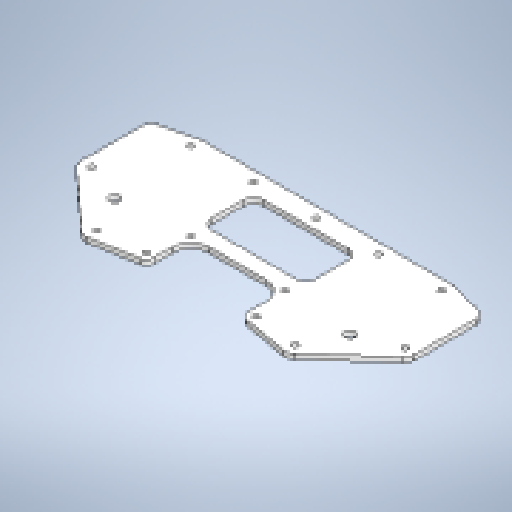
# Autodesk Inventor part: Chassis
Saved by Autodesk Inventor 2023.1 (Build 271208000, 208)
## iProperties
Created: 2022-05-26
Part Number: Chassis
Material: UHMW, White
Document SubType Name: Modeling
Designer: Nathan Cai
Density: 0.94 g/cm^3
Appearance: Smooth - White
Mass: 17.5924 g
Surface Area: 250.439 cm^2
Volume: 18.7153 cm^3
Author: Nathan Cai
Autodesk Inventor part; units mm, degrees
ref_plane "YZ Plane" through (0, 0, 0) normal (1, 0, 0) x (0, 1, 0)
ref_plane "XZ Plane" through (0, 0, 0) normal (0, 1, 0) x (-1, 0, 0)
ref_plane "XY Plane" through (0, 0, 0) normal (0, 0, 1) x (1, 0, 0)
sketch "Sketch1" plane through (0, 0, 0) normal (0, 1, 0) x (-1, 0, 0)
  line L0 (101.6, 38.1) -> (-101.6, 38.1) construction
  line L1 (-101.6, 38.1) -> (-101.6, -38.1) construction
  line L2 (-101.6, -38.1) -> (101.6, -38.1) construction
  line L3 (101.6, -38.1) -> (101.6, 38.1) construction
  line L4 (101.6, 38.1) -> (-101.6, -38.1) construction
  line L5 (-101.6, 38.1) -> (101.6, -38.1) construction
  line L6 (-28.575, 66.675) -> (28.575, 66.675) construction
  line L7 (28.575, 66.675) -> (28.575, 9.525)
  line L8 (28.575, 9.525) -> (-28.575, 9.525) construction
  line L9 (-28.575, 9.525) -> (-28.575, 66.675)
  line L10 (-28.575, 66.675) -> (28.575, 9.525) construction
  line L11 (28.575, 66.675) -> (-28.575, 9.525) construction
  circle A0 centre (-38.1, 50.8) radius 3.175
  line L12 (0, 38.1) -> (0, -38.1) construction
  circle A1 centre (-38.1, 50.8) radius 9.525
  line L13 (-38.1, 60.325) -> (-28.575, 60.325)
  circle A2 centre (38.1, 50.8) radius 3.175
  circle A3 centre (38.1, 50.8) radius 9.525
  line L14 (38.1, 60.325) -> (28.575, 60.325)
  circle A4 centre (-76.2, -38.1) radius 1.7526
  circle A5 centre (-95.25, 3.175) radius 1.7526
  circle A6 centre (76.2, -38.1) radius 1.7526
  circle A7 centre (95.25, 3.175) radius 1.7526
  line L15 (-101.6, -38.1) -> (-101.6, 6.35)
  line L16 (-101.6, 6.35) -> (-44.4797, 57.8728)
  line L17 (101.6, -38.1) -> (101.6, 6.35)
  line L18 (101.6, 6.35) -> (44.4797, 57.8728)
  line L19 (-42.6417, 42.4275) -> (-87.975, 1.5367) construction
  line L20 (-87.975, 1.5367) -> (-87.975, -38.1)
  line L21 (87.975, -38.1) -> (87.975, 1.5367)
  line L22 (87.975, 1.5367) -> (42.6417, 42.4275) construction
  line L23 (0, -38.1) -> (-95.25, -38.1) construction
  line L24 (0, -38.1) -> (95.25, -38.1) construction
  circle A8 centre (-60.325, 35.0287) radius 1.7526
  circle A9 centre (-33.3375, 31.75) radius 1.7526
  line L25 (-38.1, 0) -> (-38.1, 41.275)
  line L26 (-38.1, 0) -> (0, 0) construction
  circle A10 centre (60.325, 35.0287) radius 1.7526
  circle A11 centre (33.3375, 31.75) radius 1.7526
  line L27 (38.1, 0) -> (38.1, 41.275)
  line L28 (38.1, 0) -> (0, 0) construction
  line L29 (-87.975, 0) -> (-65.115, 0)
  line L30 (-65.115, 0) -> (-65.115, -31.75)
  line L31 (-65.115, -31.75) -> (-87.975, -31.75)
  line L32 (-101.6, -38.1) -> (101.6, -38.1) construction
  line L33 (101.6, -38.1) -> (101.6, 19.05)
  line L34 (101.6, 19.05) -> (-101.6, 19.05) construction
  line L35 (-101.6, 19.05) -> (-101.6, -38.1)
  line L36 (-101.6, 19.05) -> (-87.5203, 19.05) construction
  line L37 (87.5203, 19.05) -> (101.6, 19.05) construction
  circle A12 centre (-38.1, 0) radius 3.175 construction
  circle A13 centre (-38.1, 0) radius 6.35 construction
  circle A14 centre (38.1, 0) radius 3.175 construction
  circle A15 centre (38.1, 0) radius 6.35 construction
  circle A16 centre (28.575, 9.525) radius 1.7526
  circle A17 centre (28.575, 9.525) radius 4.7625
  arc A18 (17.0773, 9.525) -> (28.575, 21.0227) centre (17.0773, 21.0227) ccw
  circle A19 centre (-28.575, 9.525) radius 1.7526
  circle A20 centre (-28.575, 9.525) radius 4.7625
  arc A21 (-28.575, 21.0227) -> (-17.0773, 9.525) centre (-17.0773, 21.0227) ccw
  arc A22 (31.4325, 5.715) -> (38.1, 19.05) centre (21.4312, 19.05) ccw
  arc A23 (-38.1, 19.05) -> (-31.4325, 5.715) centre (-21.4312, 19.05) ccw
  line L38 (-61.94, -38.1) -> (-61.94, 25.0204)
  line L39 (87.975, 0) -> (65.115, 0)
  line L40 (65.115, 0) -> (65.115, -31.75)
  line L41 (65.115, -31.75) -> (87.975, -31.75)
  line L42 (61.94, -38.1) -> (61.94, 25.0204)
  line L43 (-28.575, 4.7625) -> (28.575, 4.7625)
  line L44 (101.6, -31.75) -> (-101.6, -31.75)
  line L45 (-101.6, -31.75) -> (-101.6, -44.45) construction
  line L46 (-101.6, -44.45) -> (101.6, -44.45)
  line L47 (101.6, -44.45) -> (101.6, -31.75) construction
  circle A24 centre (0, -38.1) radius 1.7526
  circle A25 centre (38.1, -38.1) radius 1.7526
  circle A26 centre (-38.1, -38.1) radius 1.7526
  line L48 (101.6, -38.1) -> (76.2, -44.45)
  line L49 (-101.6, -38.1) -> (-76.2, -44.45)
  line L50 (76.2, -38.1) -> (76.2, -44.45) construction
  line L51 (-76.2, -38.1) -> (-76.2, -44.45) construction
  line L52 (59.1924, 41.2769) -> (32.488, 36.4361)
  circle A27 centre (60.325, 35.0287) radius 6.35
  circle A28 centre (33.3375, 31.75) radius 4.7625
  line L53 (-59.1924, 41.2769) -> (-32.488, 36.4361)
  circle A29 centre (-60.325, 35.0287) radius 6.35
  circle A30 centre (-33.3375, 31.75) radius 4.7625
  line L54 (-87.975, 0) -> (-65.115, 0)
  line L55 (-65.115, 0) -> (-65.115, -3.175)
  line L56 (-65.115, -3.175) -> (-87.975, -3.175)
  line L57 (-87.975, -3.175) -> (-87.975, 0)
  line L58 (-65.115, -15.875) -> (-87.975, -15.875) construction
  line L59 (-65.115, -28.575) -> (-87.975, -28.575)
  line L60 (-84.8, -38.1) -> (-84.8, 0.1248)
  line L61 (65.115, -3.175) -> (87.975, -3.175)
  line L62 (65.115, -15.875) -> (87.975, -15.875) construction
  line L63 (65.115, -28.575) -> (87.975, -28.575)
  line L64 (84.8, -38.1) -> (84.8, 0.1248)
  line L65 (-31.75, -31.75) -> (31.75, -31.75)
  line L66 (31.75, -31.75) -> (31.75, 0)
  line L67 (31.75, 0) -> (-31.75, 0)
  line L68 (-31.75, 0) -> (-31.75, -31.75)
  circle A31 centre (71.465, 12.7) radius 3.175
  circle A32 centre (-71.465, 12.7) radius 3.175
  line L69 (-17.0773, 9.525) -> (17.0773, 9.525)
  point P0 (28.575, 38.1)
  point P1 (-28.575, 38.1)
  point P2 (28.575, 60.325)
  point P3 (44.4797, 57.8728)
  point P4 (101.6, -15.875)
  point P5 (38.1, 41.275)
  point P6 (-87.975, -31.75)
  point P7 (-101.6, 6.35)
  point P8 (101.6, 6.35)
  point P9 (31.75, 0)
  point P10 (38.1, 6.35)
  point P11 (-38.1, 6.35)
  point P12 (-31.75, 0)
  point P13 (87.975, 0)
  point P14 (61.94, 25.0204)
  point P15 (-17.0773, 9.525)
  point P16 (-28.575, 21.0227)
  point P17 (-38.1, 19.05)
  point P18 (-31.4325, 5.715)
  point P19 (-21.8502, 0)
  point P20 (21.8502, 0)
  point P21 (-25.2074, 12.8926)
  point P22 (-28.575, 14.2875)
  point P23 (-23.8125, 9.525)
  point P24 (-28.575, 50.8)
  point P25 (25.2074, 12.8926)
  point P26 (28.575, 14.2875)
  point P27 (23.8125, 9.525)
  point P28 (28.575, 50.8)
  point P29 (26.8224, 9.525)
  point P30 (28.575, 11.2776)
  point P31 (61.94, -31.75)
  point P32 (-61.94, -31.75)
  point P33 (-28.575, 31.75)
  point P34 (-64.5781, 39.7439)
  point P35 (64.5781, 39.7439)
  point P36 (28.575, 31.75)
  point P37 (-84.8, -3.175)
  point P38 (-84.8, -28.575)
  point P39 (84.8, -3.175)
  point P40 (84.8, -28.575)
  point P41 (31.75, -31.75)
  point P42 (-101.6, -31.75)
  point P43 (31.75, -31.75)
  point P44 (-26.8224, 9.525)
  point P45 (-28.575, 11.2776)
  point P46 (-39.8526, -38.1)
  point P47 (-36.3474, -38.1)
  point P48 (-1.7526, -38.1)
  point P49 (1.7526, -38.1)
  point P50 (36.3474, -38.1)
  point P51 (39.8526, -38.1)
  dimension "d0" = 203.2
  dimension "d1" = 76.2
  dimension "d4" = 57.15
  dimension "d6" = 6.35
  dimension "d7" = 38.1
  dimension "d8" = 19.05
  dimension "d10" = 3.5052
  dimension "d11" = 3.5052
  dimension "d12" = 0
  dimension "d14" = 25.4
  dimension "d15" = 6.35
  dimension "d20" = 50.8
  dimension "d21" = 41.275
  dimension "d22" = 44.45
  dimension "d24" = 12.7
  dimension "d25" = 13.625
  dimension "d26" = 12.7
  dimension "d27" = 13.625
  dimension "d31" = 3.5052
  dimension "d32" = 3.5052
  dimension "d33" = 6.35
  dimension "d34" = 31.75
  dimension "d35" = 4.7625
  dimension "d36" = 22.225
  dimension "d37" = 9.525
  dimension "d39" = 31.75
  dimension "d40" = 6.35
  dimension "d42" = 57.15
  dimension "d43" = 6.35
  dimension "d44" = 9.525
  dimension "d45" = 9.525
  dimension "d46" = 12.7
  dimension "d104" = 3.5052
  dimension "d105" = 9.525
  dimension "d106" = 3.175
  dimension "d107" = 22.86
  dimension "d123" = 88.9
  dimension "d124" = 12.7
  dimension "d125" = 3.5052
  dimension "d126" = 3.5052
  dimension "d127" = 38.1
  dimension "d128" = 28.575
  dimension "d129" = 3.175
  dimension "d130" = 3.175
  dimension "d131" = 31.75
  dimension "d132" = 31.75
  dimension "d133" = 31.75
  dimension "d135" = 6.35
  dimension "d136" = 12.7
  dimension "d137" = 9.525
  constraints: 141 end point, 45 symmetric about line, 28 centre point, 25 point on line, 17 parallel, 16 point on circle, 10 horizontal, 10 perpendicular, 10 tangent, 9 coincident, 9 midpoint, 5 vertical, 1 collinear, 32 other
  measures "d0" distance of L2.end L1.end
  measures "d1" distance between parallel lines of L0 L2
  measures "d4" distance of L7.end L8.end
  measures "d6" diameter of A0
  measures "d7" distance from line of L12 A0.centre
  measures "d8" diameter of A1
  measures "d10" diameter of A4
  measures "d11" diameter of A5
  measures "d12" distance from line of L2 L51.start
  measures "d14" distance from line of L1 L51.start
  measures "d15" distance from line of L1 A5.centre
  measures "d20" distance between parallel lines of L8 L14
  measures "d21" vertical distance of L51.start A5.centre
  measures "d22" distance of L1.end L15.end
  measures "d24" distance between parallel lines of L16 L19
  measures "d25" distance between parallel lines of L15 L20
  measures "d26" distance between parallel lines of L18 L22
  measures "d27" distance from line of point (101.6, -15.875) L21
  measures "d31" diameter of A8
  measures "d32" diameter of A9
  measures "d33" distance from line of L16 A8.centre
  measures "d34" distance from line of L9 A8.centre
  measures "d35" distance from line of L9 A9.centre
  measures "d36" distance from line of L8 A9.centre
  measures "d37" distance between parallel lines of L9 L25
  measures "d39" distance between parallel lines of L31 L29
  measures "d40" distance between parallel lines of L23 L31
  measures "d42" distance of L33.end L32.end
  measures "d43" diameter of A12
  measures "d44" distance from line of L8 A12.centre
  measures "d45" distance from line of L9 A12.centre
  measures "d46" diameter of A13
  measures "d104" diameter of A16
  measures "d105" diameter of A17
  measures "d106" distance between parallel lines of L30 L38
  measures "d107" distance between parallel lines of L20 L30
  measures "d123" distance from line of L32 A1.centre
  measures "d124" distance between parallel lines of L44 L46
  measures "d125" diameter of A24
  measures "d126" diameter of A25
  measures "d127" distance of A24.centre A25.centre
  measures "d128" distance from line of L12 A16.centre
  measures "d129" distance between parallel lines of L29 L56
  measures "d130" distance between parallel lines of L20 L60
  measures "d131" distance between parallel lines of L12 L68
  measures "d132" distance between parallel lines of L12 L66
  measures "d133" distance between parallel lines of L65 L67
  measures "d135" diameter of A31
  measures "d136" distance from line of L39 A31.centre
  measures "d137" distance from line of L42 A31.centre
extrude "Extrusion1" add sketch "Sketch1" along normal blind 3.175 contours A28 L27 A22 A17 L7 | A28 | L7 A17 A18 | L52 L27 A28 | L27 L52 A27 L18 L17 L44 L21 L39 L40 L66 L67 L68 L30 L29 L20 L15 L16 A29 L53 L25 A23 A20 L43 A17 A22 | A27 | A17 | A17 L43 A20 A21 L69 A18 | L17 L48 L46 L49 L15 L44 L31 L41 | A20 | L41 L64 L63 L21 | A23 L25 A30 L9 A20 | A20 L9 A21 | L63 L64 L61 L21 | L41 L40 L63 L64 | L61 L64 L39 L21 | L63 L40 L61 L64 | L25 L53 A30 | A30 | L61 L40 L39 L64 | A29 | L20 L59 L60 L31 | L20 L56 L60 L59 | L60 L59 L30 L31 | L20 L29 L60 L56 | L60 L56 L30 L59 | L60 L29 L30 L56
fillet "Fillet1" radius 6.35 6 edges at (101.6, 1.5875, -38.1) (101.6, 1.5875, 6.35) (-101.6, 1.5875, 6.35) (76.2, 1.5875, -44.45) (-76.2, 1.5875, -44.45) (-101.6, 1.5875, -38.1)
fillet "Fillet5" radius 6.35 4 edges at (31.75, 1.5875, 0) (-31.75, 1.5875, 0) (-31.75, 1.5875, -31.75) (31.75, 1.5875, -31.75)
equation "\"d35\" = 0.5 * d37"
body "Solid1"
